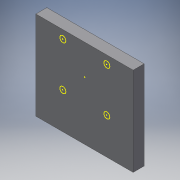
# Autodesk Inventor part: XGuideBracket
Saved by Autodesk Inventor 2019 (Build 230136000, 136)
## iProperties
Created: 2018-10-20
Part Number: XGuideBracket
Material: Generic
Document SubType Name: Modeling
Designer: LillaHunden
Density: 1 g/cm^3
Appearance: Default
Author: LillaHunden
Autodesk Inventor part; units mm, degrees
ref_plane "YZ Plane" through (0, 0, 0) normal (1, 0, 0) x (0, 1, 0)
ref_plane "XZ Plane" through (0, 0, 0) normal (0, 1, 0) x (-1, 0, 0)
ref_plane "XY Plane" through (0, 0, 0) normal (0, 0, 1) x (1, 0, 0)
sketch "Sketch1" plane through (0, 0, 0) normal (0, 0, 1) x (1, 0, 0)
  line L0 (22.0075, -26.5271) -> (-22.2094, -26.5271)
  line L1 (-22.2094, -26.5271) -> (-22.2094, 13.7173)
  line L2 (-22.2094, 13.7173) -> (22.0075, 13.7173)
  line L3 (22.0075, 13.7173) -> (22.0075, -26.5271)
  point P0 (0, 0)
  constraints: 8 end point, 2 parallel, 1 horizontal, 1 perpendicular
extrude "Extrusion1" add sketch "Sketch1" along normal blind 5
sketch "Sketch2" plane through (0, 0, 5) normal (0, 0, 1) x (1, 0, 0)
  circle A0 centre (10, -10) radius 1.35 projected
  circle A1 centre (10, 10) radius 1.375 projected
  circle A2 centre (-10, -10) radius 1.375 projected
  circle A3 centre (-10, 10) radius 1.375 projected
  point P0 (0, 0)
body "Solid1"
